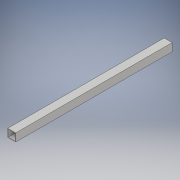
# Autodesk Inventor part: LateralBars
Saved by Autodesk Inventor 2019.3 (Build 233278000, 278)
## iProperties
Created: 2019-06-25
Part Number: LateralBars
Material: Generic
Document SubType Name: Modeling
Designer: mark
Density: 1 g/cm^3
Appearance: Default
Author: mark
Autodesk Inventor part; units mm, degrees
ref_plane "YZ Plane" through (0, 0, 0) normal (1, 0, 0) x (0, 1, 0)
ref_plane "XZ Plane" through (0, 0, 0) normal (0, 1, 0) x (-1, 0, 0)
ref_plane "XY Plane" through (0, 0, 0) normal (0, 0, 1) x (1, 0, 0)
sketch "Sketch1" plane through (0, 0, 0) normal (0, 0, 1) x (1, 0, 0)
  line L0 (10, 25.4) -> (10, 0) projected
  line L1 (35.4, 0) -> (10, 0) projected
  line L2 (35.4, 0) -> (35.4, 25.4) projected
  line L3 (35.4, 25.4) -> (10, 25.4) projected
  line L4 (125.4, 25.4) -> (125.4, 0) projected
  line L5 (150.8, 0) -> (125.4, 0) projected
  line L6 (150.8, 0) -> (150.8, 25.4) projected
  line L7 (150.8, 25.4) -> (125.4, 25.4) projected
  line L8 (10, 0) -> (35.4, 0)
  line L9 (35.4, 0) -> (35.4, 25.4)
  line L10 (35.4, 25.4) -> (10, 25.4)
  line L11 (10, 25.4) -> (10, 0)
  line L12 (11.5875, 1.5875) -> (33.8125, 1.5875)
  line L13 (33.8125, 1.5875) -> (33.8125, 23.8125)
  line L14 (33.8125, 23.8125) -> (11.5875, 23.8125)
  line L15 (11.5875, 23.8125) -> (11.5875, 1.5875)
  point P0 (0, 0)
  dimension "d0" = 22.225
  dimension "d1" = 22.225
  dimension "d2" = 1.5875
  dimension "d3" = 1.5875
  constraints: 16 end point, 4 parallel
  measures "d0" distance between parallel lines of L14 L12
  measures "d1" distance between parallel lines of L13 L15
  measures "d2" distance between parallel lines of L15 L0
  measures "d3" distance between parallel lines of L12 L1
extrude "Extrusion1" add sketch "Sketch1" along normal blind 500 contours L3 L2 L1 L0
body "Solid1"
